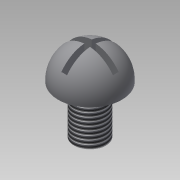
# Autodesk Inventor part: servo 4
Saved by Autodesk Inventor 2015 (Build 190159000, 159)
## iProperties
Created: 2016-07-30
Part Number: servo 4
Material: Generic
Document SubType Name: Modeling
Designer: julianesteban
Density: 1 g/cm^3
Appearance: Default
Author: julianesteban
Autodesk Inventor part; units mm, degrees
ref_plane "YZ Plane" through (0, 0, 0) normal (1, 0, 0) x (0, 1, 0)
ref_plane "XZ Plane" through (0, 0, 0) normal (0, 1, 0) x (-1, 0, 0)
ref_plane "XY Plane" through (0, 0, 0) normal (0, 0, 1) x (1, 0, 0)
sketch "Sketch1" plane through (0, 0, 0) normal (0, 0, 1) x (1, 0, 0)
  circle A0 centre (0, 0) radius 1
  dimension "d0" = 2
  constraints: 1 centre point, 1 coincident
  measures "d0" diameter of A0
extrude "Extrusion1" add sketch "Sketch1" along normal blind 3
sketch "Sketch2" plane through (0, 0, 3) normal (0, 0, 1) x (1, 0, 0)
  circle A0 centre (0, 0) radius 2
  dimension "d3" = 4
  constraints: 1 centre point, 1 coincident
  measures "d3" diameter of A0
extrude "Extrusion2" add sketch "Sketch2" along normal blind 0.1
sketch "Sketch3" plane through (0, 0, 3.1) normal (0, 0, 1) x (1, 0, 0)
  arc A0 (0, 2) -> (0, -2) centre (0, 0) ccw
  line L0 (-1.6297, -0.1797) -> (1.6297, -0.1797)
  line L1 (1.6297, -0.1797) -> (1.6297, 0.1797)
  line L2 (1.6297, 0.1797) -> (-1.6297, 0.1797)
  line L3 (-1.6297, 0.1797) -> (-1.6297, -0.1797)
  line L4 (-1.6297, -0.1797) -> (1.6297, 0.1797) construction
  line L5 (1.6297, -0.1797) -> (-1.6297, 0.1797) construction
  line L6 (0.1797, -1.6297) -> (0.1797, 1.6297)
  line L7 (0.1797, 1.6297) -> (-0.1797, 1.6297)
  line L8 (-0.1797, 1.6297) -> (-0.1797, -1.6297)
  line L9 (-0.1797, -1.6297) -> (0.1797, -1.6297)
  line L10 (0.1797, -1.6297) -> (-0.1797, 1.6297) construction
  line L11 (0.1797, 1.6297) -> (-0.1797, -1.6297) construction
  line L12 (1.6297, 0.1797) -> (-1.6297, 0.1797)
  line L13 (-1.6297, 0.1797) -> (-1.6297, -0.1797)
  line L14 (-1.6297, -0.1797) -> (1.6297, -0.1797)
  line L15 (1.6297, -0.1797) -> (1.6297, 0.1797)
  line L16 (1.6297, 0.1797) -> (-1.6297, -0.1797) construction
  line L17 (-1.6297, 0.1797) -> (1.6297, -0.1797) construction
  line L18 (-0.1797, 1.6297) -> (-0.1797, -1.6297)
  line L19 (-0.1797, -1.6297) -> (0.1797, -1.6297)
  line L20 (0.1797, -1.6297) -> (0.1797, 1.6297)
  line L21 (0.1797, 1.6297) -> (-0.1797, 1.6297)
  line L22 (-0.1797, 1.6297) -> (0.1797, -1.6297) construction
  line L23 (-0.1797, -1.6297) -> (0.1797, 1.6297) construction
  line L24 (0, 0) -> (0, 3.1525)
  line L25 (0, 3.1525) -> (0, -2)
  line L26 (0, 2) -> (0, 1.6297)
  line L27 (0, 1.6297) -> (-0.1797, 1.6297)
  line L28 (-0.1797, 1.6297) -> (-0.1797, 0.1797)
  line L29 (-0.1797, 0.1797) -> (-1.6297, 0.1797)
  line L30 (-1.6297, 0.1797) -> (-1.6297, -0.1797)
  line L31 (-1.6297, -0.1797) -> (-0.1797, -0.1797)
  line L32 (-0.1797, -0.1797) -> (-0.1797, -1.6297)
  line L33 (-0.1797, -1.6297) -> (0, -1.6297)
  line L34 (0, -1.6297) -> (0, -2)
  dimension "d8" = 360
  constraints: 70 end point, 8 point on line, 4 midpoint, 4 perpendicular, 2 collinear, 2 parallel, 2 point on circle, 1 centre point, 1 horizontal, 1 vertical, 41 other
revolve "Revolution1" add sketch "Sketch3" angle 90 about axis through (0, 3.1525, 3.1) along (0, 1, 0) contours L24 L7 L8 L2 L3 L0 L9 L25 A0
sketch "Sketch4" plane through (0, 0, 3.1) normal (0, 0, 1) x (1, 0, 0)
  line L0 (0, 0.1797) -> (-1.6297, 0.1797) projected
  line L1 (0, -0.1797) -> (-1.6297, -0.1797) projected
  line L2 (-1.6297, 0.1797) -> (-1.6297, -0.1797) projected
  line L3 (-0.1797, 1.6297) -> (-0.1797, 0.1797) projected
  line L4 (0, 1.6297) -> (-0.1797, 1.6297) projected
  line L5 (0, -1.6297) -> (0, -2) projected
  arc A0 (0, -2) -> (0, 2) centre (0, 0) ccw projected
  line L6 (0, 2) -> (0, 1.6297) projected
  line L7 (0, 1.6297) -> (-0.1797, 1.6297) projected
  line L8 (-0.1797, 1.6297) -> (-0.1797, 0.1797) projected
  line L9 (-0.1797, 0.1797) -> (-1.6297, 0.1797) projected
  line L10 (-1.6297, 0.1797) -> (-1.6297, -0.1797) projected
  line L11 (-1.6297, -0.1797) -> (-0.1797, -0.1797) projected
  line L12 (-0.1797, -0.1797) -> (-0.1797, -1.6297) projected
  line L13 (-0.1797, -1.6297) -> (0, -1.6297) projected
  line L14 (-0.1797, 1.6297) -> (0.2047, 1.6297)
  line L15 (0.2047, 1.6297) -> (0.2047, -1.6297)
  line L16 (0.2047, -1.6297) -> (-0.1797, -1.6297)
  line L17 (-0.1797, -1.6297) -> (-0.1797, 1.6297)
  line L18 (-1.6297, -0.1797) -> (1.0723, -0.1797)
  line L19 (1.0723, -0.1797) -> (1.0723, 0.2925)
  line L20 (1.0723, 0.2925) -> (-1.6297, 0.2925)
  line L21 (-1.6297, 0.2925) -> (-1.6297, -0.1797)
  constraints: 16 end point, 4 parallel, 2 horizontal, 2 perpendicular
extrude "Extrusion3" cut sketch "Sketch4" along normal blind 10 contours L17 L1 L2 L0 | L0 L21 L20 L3 | L3 L20 L15 L18 L1 L17 | L3 L4 L14 L15 L20 | L1 L18 L15 L16 L13 L12 | L20 L19 L18 L15
sketch "Sketch5" plane through (0, 0, 3.1) normal (0, 0, 1) x (1, 0, 0)
  arc A0 (0, 2) -> (0, -2) centre (0, 0) ccw
  line L0 (-1.6297, -0.1797) -> (1.6297, -0.1797)
  line L1 (1.6297, -0.1797) -> (1.6297, 0.1797)
  line L2 (1.6297, 0.1797) -> (-1.6297, 0.1797)
  line L3 (-1.6297, 0.1797) -> (-1.6297, -0.1797)
  line L4 (-1.6297, -0.1797) -> (1.6297, 0.1797) construction
  line L5 (1.6297, -0.1797) -> (-1.6297, 0.1797) construction
  line L6 (0.1797, -1.6297) -> (0.1797, 1.6297)
  line L7 (0.1797, 1.6297) -> (-0.1797, 1.6297)
  line L8 (-0.1797, 1.6297) -> (-0.1797, -1.6297)
  line L9 (-0.1797, -1.6297) -> (0.1797, -1.6297)
  line L10 (0.1797, -1.6297) -> (-0.1797, 1.6297) construction
  line L11 (0.1797, 1.6297) -> (-0.1797, -1.6297) construction
  line L12 (1.6297, 0.1797) -> (-1.6297, 0.1797)
  line L13 (-1.6297, 0.1797) -> (-1.6297, -0.1797)
  line L14 (-1.6297, -0.1797) -> (1.6297, -0.1797)
  line L15 (1.6297, -0.1797) -> (1.6297, 0.1797)
  line L16 (1.6297, 0.1797) -> (-1.6297, -0.1797) construction
  line L17 (-1.6297, 0.1797) -> (1.6297, -0.1797) construction
  line L18 (-0.1797, 1.6297) -> (-0.1797, -1.6297)
  line L19 (-0.1797, -1.6297) -> (0.1797, -1.6297)
  line L20 (0.1797, -1.6297) -> (0.1797, 1.6297)
  line L21 (0.1797, 1.6297) -> (-0.1797, 1.6297)
  line L22 (-0.1797, 1.6297) -> (0.1797, -1.6297) construction
  line L23 (-0.1797, -1.6297) -> (0.1797, 1.6297) construction
  line L24 (0, 0) -> (0, 3.1525)
  line L25 (0, 3.1525) -> (0, -2)
  line L26 (0, 2) -> (0, 1.6297)
  line L27 (0, 1.6297) -> (-0.1797, 1.6297)
  line L28 (-0.1797, 1.6297) -> (-0.1797, 0.1797)
  line L29 (-0.1797, 0.1797) -> (-1.6297, 0.1797)
  line L30 (-1.6297, 0.1797) -> (-1.6297, -0.1797)
  line L31 (-1.6297, -0.1797) -> (-0.1797, -0.1797)
  line L32 (-0.1797, -0.1797) -> (-0.1797, -1.6297)
  line L33 (-0.1797, -1.6297) -> (0, -1.6297)
  line L34 (0, -1.6297) -> (0, -2)
  line L35 (0, -1.6297) -> (0, -2) projected
  arc A1 (0, -2) -> (0, 2) centre (0, 0) ccw
  line L36 (0, 2) -> (0, 1.6297) projected
  line L37 (0, 1.6297) -> (-0.1797, 1.6297) projected
  line L38 (-0.1797, 1.6297) -> (-0.1797, 0.2925) projected
  line L39 (-0.1797, 0.2925) -> (-1.6297, 0.2925) projected
  line L40 (-1.6297, 0.2925) -> (-1.6297, -0.1797) projected
  line L41 (-1.6297, -0.1797) -> (-0.1797, -0.1797) projected
  line L42 (-0.1797, -0.1797) -> (-0.1797, -1.6297) projected
  line L43 (-0.1797, -1.6297) -> (0, -1.6297) projected
  line L44 (0, 2) -> (0, 1.6297)
  line L45 (0, 1.6297) -> (0.1797, 1.6297)
  line L46 (0.1797, 1.6297) -> (0.1797, 0.1797)
  line L47 (0.1797, 0.1797) -> (1.6297, 0.1797)
  line L48 (1.6297, 0.1797) -> (1.6297, -0.1797)
  line L49 (1.6297, -0.1797) -> (0.1797, -0.1797)
  line L50 (0.1797, -0.1797) -> (0.1797, -1.6297)
  line L51 (0.1797, -1.6297) -> (0, -1.6297)
  line L52 (0, -1.6297) -> (0, -2)
  line L53 (0, -2) -> (0, -1.6297) projected
  dimension "d15" = 360
  constraints: 88 end point, 12 point on line, 7 collinear, 5 perpendicular, 4 midpoint, 4 point on circle, 2 centre point, 2 parallel, 2 vertical, 1 horizontal, 41 other
revolve "Revolution2" add sketch "Sketch5" angle 90 about axis through (0, 3.1525, 3.1) along (0, -1, 0) contours A1 L25 L9 L6 L0 L1 L2 L7 L24
sketch "Sketch6" plane through (0, 0, 3.1) normal (0, 0, 1) x (1, 0, 0)
  circle A0 centre (0, 0) radius 1 projected
  line L0 (-0.1797, -1.6297) -> (0.1797, -1.6297) projected
  line L1 (0.1797, -1.6297) -> (0.1797, -0.1797) projected
  line L2 (0.1797, -0.1797) -> (1.6297, -0.1797) projected
  line L3 (1.6297, -0.1797) -> (1.6297, 0.1797) projected
  line L4 (1.6297, 0.1797) -> (0.1797, 0.1797) projected
  line L5 (0.1797, 0.1797) -> (0.1797, 1.6297) projected
  line L6 (0.1797, 1.6297) -> (-0.1797, 1.6297) projected
  line L7 (-0.1797, 1.6297) -> (-0.1797, 0.2925) projected
  line L8 (-0.1797, 0.2925) -> (-1.6297, 0.2925) projected
  line L9 (-1.6297, 0.2925) -> (-1.6297, -0.1797) projected
  line L10 (-1.6297, -0.1797) -> (-0.1797, -0.1797) projected
  line L11 (-0.1797, -0.1797) -> (-0.1797, -1.6297) projected
extrude "Extrusion4" cut sketch "Sketch6" along normal blind 10 contours A0 L2 L1 L11 L10 L8 L7 L5 L4 | A0 L4 L3 L2 | A0 L7 L6 L5 | L1 L0 L11 A0 | A0 L10 L9 L8
thread "Thread1" size "M2x0.25" class "6g" standard "ANSI Metric M Profile" full length
body "Solid1"
